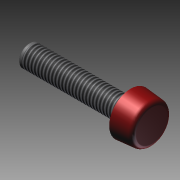
# Autodesk Inventor part: 305208-KOMP
Saved by Autodesk Inventor 2011 SP1 (Build 150282100, 282)
## iProperties
Created: 2018-01-28
Part Number: 305208-KOMP
Catalog Web Link: www.cadenas.de
Description: 305208-KOMP-U-Spannarm
Vendor: DESTACO
Document SubType Name: Modeling
Designer: psAdmin
Manufacturer: DESTACO
Mass: 0.824394 g
Surface Area: 6.57076 cm^2
Volume: 0.824394 cm^3
Density: 1 g/cm^3
Category: PARTsolutions
Company: DESTACO
Title: 305208-KOMP
Author: Cadenas PARTsolutions
Comments: U-Spannarm
PSOL_IDENT_0: {$CADENAS_DATA\23d-libs\destaco\destaco_gmbh\man_spann\horizontalspanner\kompakt\u_kompakt_parts\and
PSOL_IDENT_1: ruckspindel_u_komp.prj},162 {VTYP=3D},{NB=305208-KOMP},{LINA=305208-KOMP},{NN=305208-KOMP},{DATE=20.
PSOL_IDENT_2: 09.2016 07:53:11},{GEOMDATE=16.03.2006},{VERSION=v1},{LINEID=10},{LINESUBID=-1},{WBVAR=}  {NB=305208
PSOL_IDENT_3: -KOMP},{LINA=305208-KOMP},{KT=DUMMY},{MODELL=305208-KOMP},{SIZE=1.000}
NN: 305208-KOMP
NT: U-Spannarm
NB: 305208-KOMP
NBSYN: $MODELL.
LINA: 305208-KOMP
MODELL: 305208-KOMP
SIZE: 1.000
SUPPLIER: DESTACO
ARTICLENO: 305208-KOMP
BOMINFO: 305208-KOMP
CREATOR: CADENAS GmbH
Autodesk Inventor part; units mm, degrees
sketch "Skizze_1" plane through (0, 0, 0) normal (0, 1, 0) x (-1, 0, 0)
  line L0 (-29, 0) -> (0, 0)
  line L1 (0, 0) -> (0, -2.067)
  line L2 (0, -2.067) -> (-0.433, -2.5)
  line L3 (-0.433, -2.5) -> (-24, -2.5)
  line L4 (-24, -2.5) -> (-24, -5)
  line L5 (-24, -5) -> (-28.0872, -4.6424)
  arc A0 (-29, -3.6462) -> (-28.0872, -4.6424) centre (-28, -3.6462) ccw
  line L6 (-29, -3.6462) -> (-29, 0)
  line L7 (-29, 0) -> (0, 0)
  constraints: 16 end point, 2 point on circle, 1 centre point
revolve "Revolution1" add sketch "Skizze_1" angle 360 about axis through (29, 0, 0) along (1, 0, 0)
thread "Thread1" size "M5x0.8" class "6g" standard "ISO Metric profile" length 23.5 offset 0.5
ref_plane "AS_XY" through (12.5, 0, 0) normal (1, 0, 0) x (0, 0, -1)
ref_plane "AS_YZ" through (12.5, 0, 0) normal (0, 0, -1) x (0, 1, 0)
ref_plane "AS_ZX" through (12.5, 0, 0) normal (0, 1, 0) x (1, 0, 0)
body "Solid1"
